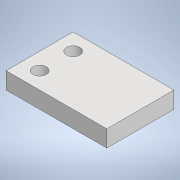
# Autodesk Inventor part: Mount_Frame
Saved by Autodesk Inventor 2022 (Build 260153070, 153G)
## iProperties
Created: 2022-03-06
Part Number: Mount_Frame
Material: Generic
Document SubType Name: Modeling
Designer: a laptop
Density: 1 g/cm^3
Appearance: Default
Author: a laptop
Autodesk Inventor part; units mm, degrees
ref_plane "YZ Plane" through (0, 0, 0) normal (1, 0, 0) x (0, 1, 0)
ref_plane "XZ Plane" through (0, 0, 0) normal (0, 1, 0) x (-1, 0, 0)
ref_plane "XY Plane" through (0, 0, 0) normal (0, 0, 1) x (1, 0, 0)
sketch "Sketch1" plane through (0, 0, 0) normal (0, 1, 0) x (-1, 0, 0)
  circle A0 centre (0, 10) radius 4
  circle A1 centre (0, -10) radius 4
  line L0 (10, 20) -> (-50, 20)
  line L1 (-50, 20) -> (-50, -20)
  line L2 (-50, -20) -> (10, -20)
  line L3 (10, -20) -> (10, 20)
  line L4 (0, 10) -> (0, -10)
  point P0 (0, 0)
  point P1 (0, 0)
  dimension "d0" = 8
  dimension "d1" = 40
  dimension "d2" = 20
  dimension "d3" = 10
  constraints: 10 end point, 2 centre point, 2 coincident, 2 parallel, 1 equal radius, 1 horizontal, 1 midpoint, 1 perpendicular, 1 vertical, 1 vertical alignment
  measures "d0" diameter of A0
  measures "d1" distance of L2.end L0.start
  measures "d2" distance of L4.end L4.start
  measures "d3" distance from line of L3 L4.start
extrude "Extrusion1" add sketch "Sketch1" along normal blind 10
sketch "Sketch2" plane through (50, 0, -20) normal (0, 0, -1) x (-1, 0, 0)
  circle A0 centre (-12, -60) radius 57.5 construction
  line L0 (0, 0) -> (60, 0) projected
  line L1 (0, 0) -> (-23.9149, -54.8004)
  line L2 (-0.0851, -65.1996) -> (28.3679, 0)
  circle A1 centre (-12, -60) radius 9 construction
  circle A2 centre (-4.2058, -64.5) radius 1.5
  circle A3 centre (-19.7942, -64.5) radius 1.5
  circle A4 centre (-12, -51) radius 1.5
  circle A5 centre (-12, -60) radius 13
  line L3 (-19.7942, -64.5) -> (-4.2058, -64.5) construction
  line L4 (-12, -51) -> (-4.2058, -64.5) construction
  line L5 (-19.7942, -64.5) -> (-12, -51) construction
  arc A6 (33.3679, 0) -> (24.0722, -9.8435) centre (42.4028, -17.843) ccw
  line L6 (0, 0) -> (0, 10)
  line L7 (-19.4144, -70.6783) -> (44, -114.7095)
  line L8 (44, -114.7095) -> (54, -114.7095)
  line L9 (54, -114.7095) -> (54, -90)
  line L10 (54, -90) -> (-4.5856, -49.3217)
  line L11 (0, 0) -> (0, 10) projected
  arc A7 (8.1288, -46.3777) -> (12.283, -61.0342) centre (19.1271, -51.1773) ccw
  circle A8 centre (-12, -60) radius 6
  point P0 (50, 0)
  point P1 (4.1861, -55.4122)
  dimension "d6" = 115
  dimension "d7" = 3
  dimension "d8" = 18
  dimension "d9" = 26
  dimension "d10" = 60
  dimension "d11" = 12
  dimension "d12" = 5
  dimension "d13" = 20
  dimension "d15" = 66
  dimension "d18" = 10
  dimension "d19" = 30
  dimension "d20" = 12
  dimension "d21" = 12
  constraints: 20 end point, 11 point on circle, 9 centre point, 7 tangent, 5 point on line, 3 coincident, 2 equal length, 2 equal radius, 2 horizontal, 2 parallel, 1 perpendicular
  measures "d6" diameter of A0
  measures "d7" diameter of A4
  measures "d8" diameter of A1
  measures "d9" diameter of A5
  measures "d10" vertical distance of L0.start A0.centre
  measures "d11" horizontal distance of L0.start A0.centre
  measures "d12" distance of L2.end A6.start
  measures "d13" radius of A6
  measures "d15" horizontal distance of A0.centre L9.end
  measures "d18" distance of L7.end L8.end
  measures "d19" vertical distance of A0.centre L9.end
  measures "d20" radius of A7
  measures "d21" diameter of A8
extrude "Extrusion2" add sketch "Sketch2" against normal blind 10
sketch "Sketch3" plane through (50, 0, -10) normal (0, 0, 1) x (1, 0, 0)
  circle A0 centre (-49, -95.3547) radius 2
  circle A1 centre (-49, -109.3547) radius 2
  line L0 (-54, -90) -> (-44, -90)
  line L1 (-44, -90) -> (-44, -114.7095)
  line L2 (-44, -114.7095) -> (-54, -114.7095)
  line L3 (-54, -114.7095) -> (-54, -90)
  line L4 (-49, -95.3547) -> (-49, -109.3547)
  point P0 (-50, 0)
  point P1 (-44, -102.3547)
  point P2 (-49, -102.3547)
  point P3 (-49, -90)
  dimension "d24" = 4
  dimension "d25" = 14
  constraints: 11 end point, 3 midpoint, 2 centre point, 2 parallel, 2 perpendicular, 1 coincident, 1 equal radius, 1 horizontal, 1 horizontal alignment, 1 vertical alignment
  measures "d24" diameter of A1
  measures "d25" distance of L4.start L4.end
extrude "Extrusion3" cut sketch "Sketch3" against normal blind 10 contours A0 | A1
body "Solid1"
